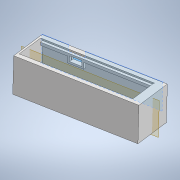
# Autodesk Inventor part: battery and buck converter enclosure
Saved by Autodesk Inventor 2022 (Build 260153000, 153)
## iProperties
Created: 2021-10-07
Part Number: battery and buck converter enclosure
Material: Generic
Document SubType Name: Modeling
Designer: tecware
Density: 1 g/cm^3
Appearance: Default
Author: tecware
## iProperties of the stored document battery and buck converter enclosure_3DPrint.ipt
Created: 2021-10-07
Part Number: battery and buck converter enclosure_3DPrint
Material: Generic
Document SubType Name: Modeling
Designer: tecware
Density: 1 g/cm^3
Appearance: Default
Author: tecware
Autodesk Inventor part; units mm, degrees
ref_plane "YZ Plane" through (0, 0, 0) normal (1, 0, 0) x (0, 1, 0)
ref_plane "XZ Plane" through (0, 0, 0) normal (0, 1, 0) x (-1, 0, 0)
ref_plane "XY Plane" through (0, 0, 0) normal (0, 0, 1) x (1, 0, 0)
sketch "Sketch1" plane through (0, 0, 0) normal (0, 1, 0) x (-1, 0, 0)
  line L0 (90, -20.5) -> (-30, -20.5)
  line L1 (-30, -20.5) -> (-30, 15.5)
  line L2 (-30, 15.5) -> (90, 15.5)
  line L3 (90, 15.5) -> (90, -20.5)
  dimension "d0" = 120
  dimension "d1" = 36
  constraints: 8 end point, 2 parallel, 1 horizontal, 1 perpendicular
  measures "d0" distance of L1.end L2.end
  measures "d1" distance of L0.end L1.end
extrude "Main Body" add sketch "Sketch1" along normal blind 35
shell "Main Shell" thickness 2 outward yes removed faces 1 at (-50, 35, 3.5)
ref_plane "Work Plane2" through (-92, -2, -2.5) normal (0, 0, 1) x (1, 0, 0)
sketch "Sketch19" plane through (-90, 0, -20.5) normal (1, 0, 0) x (0, 0, -1)
  line L0 (-36, 35) -> (-36, 31)
  line L1 (-36, 35) -> (-33, 35)
  line L2 (2, 35) -> (-38, 35) projected
  line L3 (-36, 31) -> (-33, 35)
  line L4 (-18, 35) -> (-18, 25)
  line L5 (-36, 31) -> (-33, 31)
  line L6 (-33, 31) -> (-33, 28)
  line L7 (-33, 28) -> (-36, 28)
  line L8 (-36, 28) -> (-36, 31)
  line L9 (0, 0) -> (-36, 0) projected
  line L10 (0, 0) -> (0, 35) projected
  line L11 (-36, 35) -> (0, 35) projected
  line L12 (-36, 0) -> (-36, 35) projected
  line L13 (0, 35) -> (0, 31)
  line L14 (0, 35) -> (-3, 35)
  line L15 (0, 31) -> (-3, 35)
  line L16 (0, 31) -> (-3, 31)
  line L17 (-3, 31) -> (-3, 28)
  line L18 (-3, 28) -> (0, 28)
  line L19 (0, 28) -> (0, 31)
  line L20 (-36, 35) -> (0, 35) projected
  point P0 (-20.5, 0)
  point P1 (-36, 33)
  point P2 (0, 33)
  point P3 (-3, 35)
  dimension "d107" = 3
  dimension "d108" = 4
  dimension "d109" = 3
  dimension "d110" = 3
  constraints: 30 end point, 8 symmetric about line, 3 point on line, 2 horizontal, 2 midpoint, 2 parallel, 2 vertical, 1 perpendicular
  measures "d107" distance of L0.start L1.end
  measures "d108" distance of L0.start L0.end
  measures "d109" distance of L7.end L0.end
  measures "d110" distance of L6.end L7.end
extrude "Rail" add sketch "Sketch19" along normal up to surface (122 mm away) contours L1 L3 L0 | L5 L6 L7 L8 | L2 L10 L15 | L10 L18 L17 L16
sketch "Sketch27" plane through (-92, -2, -2.5) normal (0, 0, 1) x (1, 0, 0)
  line L0 (124, 0) -> (124, 37) projected
  line L1 (122, 33) -> (2, 33) projected
  line L2 (2, 37) -> (122, 37) projected
  line L3 (122, 37) -> (122.5, 37)
  line L4 (124, 37) -> (0, 37) projected
  line L5 (122.5, 37) -> (114.5, 37)
  line L6 (118.5, 37) -> (118.5, 35)
  line L7 (118.0528, 35.2236) -> (114.5, 37)
  line L8 (118.9472, 35.2236) -> (122.5, 37)
  arc A0 (118.0528, 35.2236) -> (118.9472, 35.2236) centre (118.5, 36.118) ccw
  point P0 (92, 2)
  dimension "d157" = 0.5
  dimension "d158" = 8
  dimension "d159" = 2
  dimension "d160" = 1
  constraints: 10 end point, 4 point on line, 2 point on circle, 2 tangent, 1 centre point, 1 midpoint, 1 vertical
  measures "d157" distance of L2.end L3.end
  measures "d158" distance of L3.end L5.end
  measures "d159" distance of L6.start L6.end
  measures "d160" radius of A0
extrude "Groove for snap fit" add sketch "Sketch27" along normal mid plane 39
sketch "Sketch28" plane through (30, 0, -20.5) normal (-1, 0, 0) x (0, 0, 1)
  line L0 (3, 27) -> (0, 27)
  line L1 (0, 27) -> (0, 30)
  line L2 (0, 30) -> (3, 30)
  line L3 (3, 30) -> (3, 27)
  line L4 (33.1875, 34.75) -> (2.8125, 34.75) projected
  line L5 (18, 34.75) -> (18, 27.43)
  line L6 (33, 27) -> (36, 27)
  line L7 (36, 27) -> (36, 30)
  line L8 (36, 30) -> (33, 30)
  line L9 (33, 30) -> (33, 27)
  point P0 (20.5, 0)
  constraints: 18 end point, 4 symmetric about line, 2 parallel, 1 horizontal, 1 midpoint, 1 perpendicular, 1 vertical
extrude "Groove corner fill (redundant)" [suppressed]
fillet "Fillet3" radius 0.75 1 edges at (30, 34.75, -2.5)
sketch "Sketch3" plane through (-90, 0, -20.5) normal (0, 0, 1) x (1, 0, 0)
  line L0 (28.9, 29) -> (41.1, 29)
  line L1 (41.1, 29) -> (41.1, 23.5)
  line L2 (41.1, 23.5) -> (28.9, 23.5)
  line L3 (28.9, 23.5) -> (28.9, 29)
  line L4 (0, 35) -> (120, 35) projected
  point P0 (90, 0)
  dimension "d9" = 12.2
  dimension "d10" = 5.5
  dimension "d75" = 6
  constraints: 8 end point, 2 parallel, 1 horizontal, 1 perpendicular
  measures "d9" distance of L1.end L2.end
  measures "d10" distance of L0.end L1.end
  measures "d75" distance between parallel lines of L4 L0
extrude "Switch Cutout" cut sketch "Sketch3" along normal mid plane 16
sketch "Sketch8" plane through (-90, 0, -20.5) normal (0, 0, 1) x (1, 0, 0)
  line L0 (28.9, 23.5) -> (41.1, 23.5) projected
  line L1 (29, 35.5) -> (41.1, 35.5)
  line L2 (41.1, 35.5) -> (41.1, 23.5)
  line L3 (41.1, 23.5) -> (29, 23.5)
  line L4 (29, 23.5) -> (29, 35.5)
  line L5 (27, 35.5) -> (43.1, 35.5)
  line L6 (43.1, 35.5) -> (43.1, 21.5)
  line L7 (43.1, 21.5) -> (27, 21.5)
  line L8 (27, 21.5) -> (27, 35.5)
  line L9 (27, 29) -> (43.1, 29)
  point P0 (90, 0)
  point P1 (29, 23.5)
  point P2 (41.1, 29)
  point P3 (29, 29)
  dimension "d40" = 2
  dimension "d41" = 2
  dimension "d42" = 2
  dimension "d77" = 5.5
  constraints: 18 end point, 4 parallel, 3 perpendicular, 2 horizontal, 2 point on line
  measures "d40" distance between parallel lines of L4 L8
  measures "d41" distance between parallel lines of L6 L2
  measures "d42" distance between parallel lines of L0 L7
  measures "d77" distance between parallel lines of L9 L0
extrude "Switch Holder" add sketch "Sketch8" along normal blind 3 contours L0 L2 L9 L6 L7 L8 L4
sketch "Sketch35" plane through (-90, 0, -20.5) normal (0, 0, 1) x (1, 0, 0)
  line L0 (41.1, 23.5) -> (41.1, 29) projected
  line L1 (41.1, 26.25) -> (68.4762, 26.25) construction
  line L2 (43.1, 28) -> (55.1, 28)
  line L3 (55.1, 28) -> (55.1, 16)
  line L4 (55.1, 16) -> (43.1, 16)
  line L5 (43.1, 16) -> (43.1, 28)
  circle A0 centre (49.1, 22) radius 3.5
  point P0 (90, 0)
  point P1 (43.1, 21.5)
  dimension "d205" = 12
  dimension "d206" = 12
  dimension "d207" = 7
  constraints: 10 end point, 2 horizontal, 2 parallel, 1 centre point, 1 midpoint, 1 perpendicular
  measures "d205" distance of L3.end L4.end
  measures "d206" distance of L2.end L3.end
  measures "d207" diameter of A0
extrude "Extrusion18" cut sketch "Sketch35" against normal blind 10 contours A0
sketch "Sketch9" plane through (-92, -2, -22.5) normal (-1, 0, 0) x (0, 0, 1)
  circle A0 centre (20, 18.5) radius 6
  circle A1 centre (20, 18.5) radius 8
  line L0 (38, 2) -> (38, 37) projected
  line L1 (2, 2) -> (38, 2) projected
  point P0 (22.5, 2)
  dimension "d45" = 12
  dimension "d46" = 16
  dimension "d78" = 18
  dimension "d79" = 16.5
  constraints: 2 centre point, 1 coincident
  measures "d45" diameter of A0
  measures "d46" diameter of A1
  measures "d78" distance from line of L0 A0.centre
  measures "d79" distance from line of L1 A0.centre
extrude "Raised" add sketch "Sketch9" along normal blind 2.2
sketch "thread" plane through (-94.2, 3.5, -20) normal (-1, 0, 0) x (0, 0, 1)
  circle A0 centre (17.5, 13) radius 6
  circle A1 centre (17.5, 13) radius 10
  line L0 (35.5, -3.5) -> (35.5, 24.5) projected
  line L1 (-0.5, -3.5) -> (35.5, -3.5) projected
  point P0 (20, -3.5)
  dimension "d13" = 12
  dimension "d14" = 20
  dimension "d135" = 18
  dimension "d136" = 16.5
  constraints: 2 centre point, 2 coincident
  measures "d13" diameter of A0
  measures "d14" diameter of A1
  measures "d135" distance from line of L0 A0.centre
  measures "d136" distance from line of L1 A0.centre
extrude "For Threads" add sketch "thread" along normal blind 10 contours A0 | A1
sketch "Sketch13" plane through (-90, 15, -5) normal (-1, 0, 0) x (0, 0, 1)
  circle A0 centre (2.5, 1.5) radius 6
  line L0 (-15.5, -15) -> (-15.5, 13) projected
  line L1 (-15.5, -15) -> (20.5, -15) projected
  line L2 (20.5, -15) -> (20.5, 13) projected
  point P0 (5, -15)
  dimension "d72" = 12
  dimension "d137" = 18
  dimension "d138" = 16.5
  constraints: 1 centre point
  measures "d72" diameter of A0
  measures "d137" distance from line of L2 A0.centre
  measures "d138" distance from line of L1 A0.centre
extrude "Through Hole For Wire" cut sketch "Sketch13" along normal through all
sketch "Sketch23" plane through (-90, 0, 15.5) normal (1, 0, 0) x (0, 0, -1)
  circle A0 centre (18, 16.5) radius 6 projected
  line L0 (3, 28) -> (0, 28) projected
  line L1 (0, 0) -> (0, 28) projected
  line L2 (36, 0) -> (0, 0) projected
  line L3 (36, 0) -> (36, 28) projected
  line L4 (36, 28) -> (33, 28) projected
  line L5 (33, 28) -> (33, 31) projected
  line L6 (33, 31) -> (36, 31) projected
  line L7 (36, 31) -> (33, 35) projected
  line L8 (3, 35) -> (33, 35) projected
  line L9 (3, 35) -> (0, 31) projected
  line L10 (0, 31) -> (3, 31) projected
  line L11 (3, 31) -> (3, 28) projected
  line L12 (3, 31) -> (3, 28) projected
  line L13 (3, 31) -> (33, 31)
  line L14 (33, 28) -> (33, 31) projected
  line L15 (33, 30) -> (3, 30)
  point P0 (15.5, 0)
  point P1 (3, 30)
  dimension "d185" = 1
  constraints: 4 end point, 2 perpendicular, 2 point on line
  measures "d185" distance between parallel lines of L13 L15
extrude "Cutout for cover" cut sketch "Sketch23" against normal up to next contours L10 L9 L8 L7 L6 L13
fillet "Fillet1" radius 4 4 edges at (-30, 35, 17.5) (-30, 35, -22.5) (-30, -2, 17.5) (-30, -2, -22.5)
thread "Thread5" size "M22x3" class "6g" standard "ANSI Metric M Profile" full length
equation "\"d41\" = d40"
equation "\"d42\" = d40"
equation "\"d77\" = d10"
equation "\"d78\" = 0.5 * d1"
equation "\"d79\" = -0.5 * d8 + 0.5 * d2"
equation "\"d135\" = d78"
equation "\"d136\" = d79"
equation "\"d137\" = d78"
equation "\"d138\" = d79"
equation "\"d28\" = 55deg"
equation "\"Sketch5_Pitch\" = 3"
equation "\"d60\" = 55deg"
equation "\"Sketch10_Pitch\" = 3"
equation "\"d91\" = 55deg"
equation "\"Sketch14_Pitch\" = 3"
equation "\"d123\" = 55deg"
equation "\"Sketch20_Pitch\" = 3"
equation "\"d173\" = 55deg"
equation "\"Sketch29_Pitch\" = 3"
equation "\"d193\" = 55deg"
equation "\"Sketch32_Pitch\" = 3"
equation "\"d8\" = 2"
equation "\"d2\" = 35"
body "Solid1"
